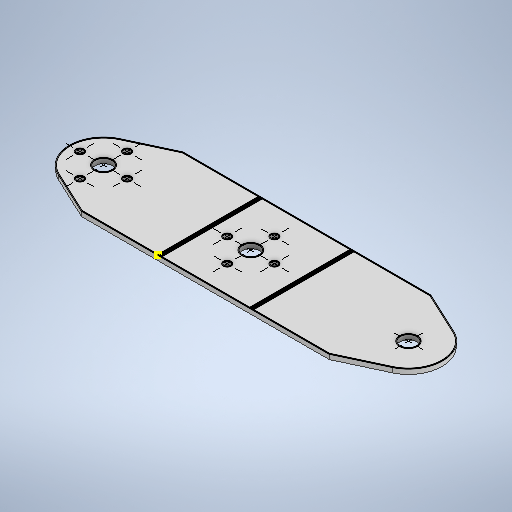
# Autodesk Inventor part: CAM_axis_1_supplement_frame
Saved by Autodesk Inventor 2025.2 (Build 292293000, 293)
## iProperties
Created: 2025-08-09
Part Number: CAM_axis_1_supplement_frame
Material: Generic
Document SubType Name: Modeling
Designer: User
Density: 1 g/cm^3
Appearance: Default
Author: User
Autodesk Inventor part; units mm, degrees
ref_plane "YZ Plane" through (0, 0, 0) normal (1, 0, 0) x (0, 1, 0)
ref_plane "XZ Plane" through (0, 0, 0) normal (0, 1, 0) x (-1, 0, 0)
ref_plane "XY Plane" through (0, 0, 0) normal (0, 0, 1) x (1, 0, 0)
sketch "Sketch1" plane through (0, 0, 0) normal (0, 1, 0) x (-1, 0, 0)
  line L0 (-27.6589, 0) -> (-27.6589, -30)
  line L1 (-0.4496, -30) -> (-0.4496, 0)
  circle A0 centre (-12.5193, -15) radius 2.6
  circle A1 centre (-5.5193, -15) radius 1.05
  circle A2 centre (-12.5193, -8) radius 1.05
  circle A3 centre (-19.5193, -15) radius 1.05
  circle A4 centre (-12.5193, -22) radius 1.05
  circle A5 centre (-59.2986, -15) radius 2.55
  circle A6 centre (31.19, -15) radius 2.6
  circle A7 centre (24.19, -15) radius 1.05
  circle A8 centre (31.19, -8) radius 1.05
  circle A9 centre (31.19, -22) radius 1.05
  circle A10 centre (38.19, -15) radius 1.05
  line L2 (35.4177, -5.9376) -> (22.69, 0)
  line L3 (-50.7986, 0) -> (-63.5263, -5.9376)
  line L4 (22.69, -30) -> (35.4177, -24.0624)
  line L5 (-63.5263, -24.0624) -> (-50.7986, -30)
  arc A11 (35.4177, -24.0624) -> (35.4177, -5.9376) centre (31.19, -15) ccw
  arc A12 (-63.5263, -5.9376) -> (-63.5263, -24.0624) centre (-59.2986, -15) ccw
  line L6 (-50.7986, 0) -> (22.69, 0)
  line L7 (22.69, -30) -> (-50.7986, -30)
  line L8 (-28.1086, -30) -> (-28.1086, 0)
  line L9 (-27.2093, 0) -> (-27.2093, -30)
  line L10 (-0.8993, -30) -> (-0.8993, 0)
  line L11 (0, 0) -> (0, -30)
  point P0 (0, 0)
  constraints: 24 end point, 13 centre point, 12 point on line, 9 equal radius, 7 parallel, 6 vertical, 4 point on circle, 4 tangent, 2 horizontal, 2 perpendicular, 49 other
extrude "Extrusion1" add sketch "Sketch1" against normal blind 1.5
body "Solid1"
